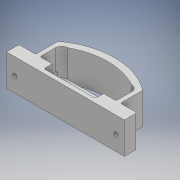
# Autodesk Inventor part: jig
Saved by Autodesk Inventor 2017 (Build 210142000, 142)
## iProperties
Part Number: jig
Material: 一般
Document SubType Name: Modeling
Designer: taige
Density: 1 g/cm^3
Appearance: 既定
Author: taige
Autodesk Inventor part; units mm, degrees
ref_plane "YZ Plane" through (0, 0, 0) normal (1, 0, 0) x (0, 1, 0)
ref_plane "XZ Plane" through (0, 0, 0) normal (0, 1, 0) x (-1, 0, 0)
ref_plane "XY Plane" through (0, 0, 0) normal (0, 0, 1) x (1, 0, 0)
sketch "スケッチ1" plane through (0, 0, 0) normal (0, 0, 1) x (1, 0, 0)
  line L0 (51, 14.4226) -> (51, -10.5774)
  line L1 (-51, -10.5774) -> (-51, 14.4226)
  circle A0 centre (-22.5, -0.0774) radius 1.6
  circle A1 centre (22.5, -0.0774) radius 1.6
  line L2 (-71, -27.5774) -> (71, -27.5774)
  line L3 (71, -27.5774) -> (71, -14.5774)
  line L4 (-53, -12.5774) -> (-69, -12.5774)
  line L5 (-71, -14.5774) -> (-71, -27.5774)
  arc A2 (-53, -12.5774) -> (-51, -10.5774) centre (-53, -10.5774) ccw
  line L6 (69, -12.5774) -> (53, -12.5774)
  arc A3 (51, -10.5774) -> (53, -12.5774) centre (53, -10.5774) ccw
  line L7 (-51, 14.4226) -> (51, 14.4226)
  arc A4 (-69, -12.5774) -> (-71, -14.5774) centre (-69, -14.5774) ccw
  arc A5 (71, -14.5774) -> (69, -12.5774) centre (69, -14.5774) ccw
  arc A6 (51, 14.4226) -> (-51, 14.4226) centre (0, -53.5774) ccw
  point P0 (0, 0)
  point P1 (0, -100)
  point P2 (71, -12.5774)
  point P3 (-71, -12.5774)
  point P4 (0, 31.4226)
  dimension "d5" = 51
  dimension "d8" = 3.2
  dimension "d10" = 3.2
  dimension "d28" = 45
  dimension "d31" = 28.5
  dimension "d35" = 142
  dimension "d36" = 15
  dimension "d38" = 2
  dimension "d39" = 2
  dimension "d42" = 20
  dimension "d47" = 100
  dimension "d48" = 51
  dimension "d55" = 102
  dimension "d56" = 42
  dimension "d57" = 2
  dimension "d58" = 2
  dimension "d73" = 27.5
  dimension "d75" = 27.5
  dimension "d76" = 17
  dimension "d86" = 20
  constraints: 16 end point, 11 point on circle, 8 tangent, 7 centre point, 5 point on line, 3 parallel, 2 horizontal, 2 perpendicular
  measures "d5" distance from line of L1 point (0, 0)
  measures "d8" diameter of A0
  measures "d10" diameter of A1
  measures "d28" distance of A0.centre A1.centre
  measures "d31" distance from line of L0 A1.centre
  measures "d35" distance of point (-71, -12.577) point (71, -12.577)
  measures "d36" distance of point (71, -12.577) L2.end
  measures "d38" radius of A2
  measures "d39" radius of A3
  measures "d42" distance between parallel lines of L3 L0
  measures "d47" distance of point (0, -100) point (0, 0)
  measures "d48" distance from line of point (0, -100) L1
  measures "d55" distance between parallel lines of L0 L1
  measures "d56" distance from line of L1.end L2
  measures "d57" radius of A4
  measures "d58" radius of A5
  measures "d73" distance from line of A0.centre L2
  measures "d75" distance from line of A1.centre L2
  measures "d76" distance from line of L7 point (0, 31.423)
  measures "d86" distance between parallel lines of L5 L1
extrude "押し出し1" add sketch "スケッチ1" along normal blind 38
sketch "スケッチ2" plane through (0, 0, 38) normal (0, 0, 1) x (1, 0, 0)
  line L0 (-39, 13.4226) -> (39, 13.4226)
  line L1 (46, 6.4226) -> (46, -10.5774)
  line L2 (44, -12.5774) -> (-44, -12.5774)
  line L3 (-46, -10.5774) -> (-46, 6.4226)
  arc A0 (-39, 13.4226) -> (-46, 6.4226) centre (-39, 6.4226) ccw
  arc A1 (46, 6.4226) -> (39, 13.4226) centre (39, 6.4226) ccw
  arc A2 (-46, -10.5774) -> (-44, -12.5774) centre (-44, -10.5774) ccw
  arc A3 (44, -12.5774) -> (46, -10.5774) centre (44, -10.5774) ccw
  circle A4 centre (22.5, -0.0774) radius 1.6 projected
  point P0 (0, 0)
  point P1 (-46, 13.4226)
  point P2 (46, -12.5774)
  point P3 (46, 13.4226)
  point P4 (-46, -12.5774)
  dimension "d17" = 92
  dimension "d18" = 26
  dimension "d19" = 46
  dimension "d23" = 7
  dimension "d24" = 7
  dimension "d25" = 2
  dimension "d26" = 2
  dimension "d50" = 12.5
  constraints: 8 end point, 8 point on circle, 8 point on line, 8 tangent, 4 centre point, 2 parallel, 1 horizontal, 1 perpendicular
  measures "d17" distance of point (46, -12.577) point (-46, -12.577)
  measures "d18" distance of point (46, 13.423) point (46, -12.577)
  measures "d19" distance from line of point (0, 0) L3
  measures "d23" radius of A0
  measures "d24" radius of A1
  measures "d25" radius of A2
  measures "d26" radius of A3
  measures "d50" distance from line of A4.centre L2
extrude "押し出し2" cut sketch "スケッチ2" against normal blind 33 contours L0 A1 L1 A3 L2 A2 L3 A0 | A4
sketch "スケッチ3" plane through (0, 0, 38) normal (0, 0, 1) x (1, 0, 0)
  line L0 (-39, 13.4226) -> (39, 13.4226) projected
  arc A0 (39, 13.4226) -> (-39, 13.4226) centre (0, -57.6274) ccw
  line L1 (-46, -10.5774) -> (-46, 6.4226) projected
  line L2 (44, -12.5774) -> (-44, -12.5774) projected
  line L3 (-39, 13.4226) -> (39, 13.4226)
  point P0 (0, 0)
  point P1 (0, 23.4226)
  dimension "d59" = 10
  constraints: 3 point on circle, 2 end point, 1 centre point, 1 coincident, 1 horizontal
  measures "d59" distance from line of point (0, 23.423) L0
extrude "押し出し3" cut sketch "スケッチ3" against normal blind 40
sketch "スケッチ4" plane through (0, 0, 38) normal (0, 0, 1) x (1, 0, 0)
  line L0 (-31, -12.5774) -> (31, -12.5774)
  line L1 (31, -12.5774) -> (31, -20.5774)
  line L2 (29, -22.5774) -> (-29, -22.5774)
  line L3 (-31, -20.5774) -> (-31, -12.5774)
  line L4 (-46, -10.5774) -> (-46, 6.4226) projected
  line L5 (44, -12.5774) -> (-44, -12.5774) projected
  arc A0 (-31, -20.5774) -> (-29, -22.5774) centre (-29, -20.5774) ccw
  arc A1 (29, -22.5774) -> (31, -20.5774) centre (29, -20.5774) ccw
  point P0 (0, 0)
  point P1 (31, -22.5774)
  point P2 (-31, -22.5774)
  dimension "d66" = 62
  dimension "d67" = 10
  dimension "d68" = 15
  dimension "d69" = 10
  dimension "d72" = 2
  constraints: 8 end point, 4 point on circle, 4 point on line, 4 tangent, 2 centre point, 2 parallel, 1 equal radius, 1 horizontal, 1 perpendicular
  measures "d66" distance of point (31, -22.577) point (-31, -22.577)
  measures "d67" distance of L0.end point (31, -22.577)
  measures "d68" distance between parallel lines of L3 L4
  measures "d69" distance between parallel lines of L5 L2
  measures "d72" radius of A0
extrude "押し出し4" cut sketch "スケッチ4" against normal blind 35
sketch "スケッチ5" plane through (-69, -12.5774, 0) normal (0, 1, 0) x (1, 0, 0)
  circle A0 centre (8, -18) radius 5.05
  line L0 (69, 0) -> (69, -40)
  circle A1 centre (130, -18) radius 5.05
  line L1 (18, 0) -> (18, -38) projected
  line L2 (16, -38) -> (0, -38) projected
  point P0 (-2, -38)
  dimension "d77" = 10.1
  dimension "d84" = 10
  dimension "d85" = 20
  constraints: 2 centre point, 2 end point, 1 symmetric about line, 1 vertical, 1 other
  measures "d77" diameter of A0
  measures "d84" distance from line of A0.centre L1
  measures "d85" distance from line of A0.centre L2
extrude "押し出し5" cut sketch "スケッチ5" against normal blind 5
sketch "スケッチ6" plane through (-61, -17.5774, 18) normal (0, 1, 0) x (1, 0, 0)
  line L0 (61, 18) -> (61, -20)
  line L1 (90, -20) -> (32, -20) projected
  circle A0 centre (0, 0) radius 2.6
  circle A1 centre (122, 0) radius 2.6
  line L2 (10, 18) -> (10, -20) projected
  line L3 (8, -20) -> (-8, -20) projected
  dimension "d81" = 5.2
  dimension "d87" = 10
  dimension "d88" = 20
  constraints: 2 centre point, 2 end point, 1 midpoint, 1 symmetric about line, 1 other
  measures "d81" diameter of A0
  measures "d87" distance from line of L2 A0.centre
  measures "d88" distance from line of L3 A0.centre
extrude "押し出し6" cut sketch "スケッチ6" against normal blind 10
sketch "スケッチ7" plane through (-51, -10.5774, 0) normal (-1, 0, 0) x (0, 0, 1)
  line L0 (7, 19) -> (11, 19)
  line L1 (13, 17) -> (13, 5)
  line L2 (11, 3) -> (7, 3)
  line L3 (5, 5) -> (5, 17)
  arc A0 (7, 19) -> (5, 17) centre (7, 17) ccw
  arc A1 (5, 5) -> (7, 3) centre (7, 5) ccw
  arc A2 (11, 3) -> (13, 5) centre (11, 5) ccw
  arc A3 (13, 17) -> (11, 19) centre (11, 17) ccw
  line L4 (0, 25) -> (0, 0) projected
  point P0 (0, 10.5774)
  point P1 (13, 3)
  point P2 (13, 19)
  point P3 (5, 3)
  point P4 (38, -2)
  dimension "d89" = 8
  dimension "d90" = 16
  dimension "d91" = 2
  dimension "d94" = 5
  dimension "d95" = 5
  constraints: 8 end point, 8 point on circle, 8 tangent, 6 point on line, 4 centre point, 3 equal radius, 2 parallel, 1 horizontal, 1 perpendicular
  measures "d89" distance of point (13, 3) point (5, 3)
  measures "d90" distance of point (13, 19) point (13, 3)
  measures "d91" radius of A0
  measures "d94" distance between parallel lines of L4 L3
  measures "d95" distance from line of L2 point (38, -2)
extrude "押し出し7" cut sketch "スケッチ7" against normal blind 8
